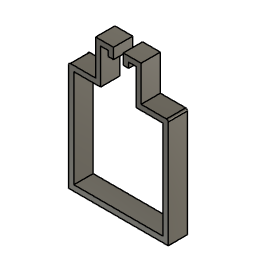
battery weight support (Autodesk Fusion 360 design; units mm, degrees)
Autodesk Fusion 360 part; units mm, degrees
sketch "Esquisse1" plane through (0, 0, 0) normal (0, 1, 0) x (1, 0, 0)
  line L0 (0, 0) -> (50, 0)
  line L1 (50, 0) -> (50, -55)
  line L2 (50, -55) -> (0, -55)
  line L3 (0, -55) -> (0, 0)
  line L4 (53, 3) -> (53, -58)
  line L5 (53, -58) -> (-3, -58)
  line L6 (-3, -58) -> (-3, 3)
  line L7 (-3, 3.2) -> (53, 3.2)
  line L8 (53, 3) -> (53, 3.2)
  line L9 (-3, 3) -> (-3, 3.2)
  line L10 (25, -55) -> (25, -58)
  line L11 (25, -58) -> (12.25, -58)
  line L12 (12.25, -58) -> (37.75, -58)
  line L13 (37.75, -58) -> (37.75, -78)
  line L14 (37.75, -78) -> (12.25, -78)
  line L15 (12.25, -78) -> (12.25, -58)
  line L16 (25, -58) -> (15, -58)
  line L17 (15, -58) -> (35, -58)
  line L18 (35, -58) -> (35, -78)
  line L19 (35, -78) -> (15, -78)
  line L20 (15, -78) -> (15, -58)
  line L21 (12.25, -58) -> (9.25, -58)
  line L22 (9.25, -58) -> (9.25, -78)
  line L23 (9.25, -78) -> (12.25, -78)
  line L24 (12.25, -78) -> (12.25, -58)
  line L25 (37.75, -58) -> (40.75, -58)
  line L26 (40.75, -58) -> (40.75, -78)
  line L27 (40.75, -78) -> (37.75, -78)
  line L28 (37.75, -78) -> (37.75, -58)
  line L29 (9.25, -78) -> (19.25, -78)
  line L30 (19.25, -78) -> (19.25, -75)
  line L31 (19.25, -75) -> (9.25, -75)
  line L32 (9.25, -75) -> (9.25, -78)
  line L33 (40.75, -78) -> (30.75, -78)
  line L34 (30.75, -78) -> (30.75, -75)
  line L35 (30.75, -75) -> (40.75, -75)
  line L36 (40.75, -75) -> (40.75, -78)
  line L37 (30.75, -75) -> (33.75, -75)
  line L38 (33.75, -75) -> (33.75, -72)
  line L39 (33.75, -72) -> (30.75, -72)
  line L40 (30.75, -72) -> (30.75, -75)
  line L41 (19.25, -75) -> (16.25, -75)
  line L42 (16.25, -75) -> (16.25, -72)
  line L43 (16.25, -72) -> (19.25, -72)
  line L44 (19.25, -72) -> (19.25, -75)
  line L45 (12.25, -58) -> (12.25, -55)
  line L46 (9.25, -58) -> (9.25, -55)
  line L47 (15, -58) -> (15, -55)
  line L48 (37.75, -58) -> (37.75, -55)
  line L49 (40.75, -58) -> (40.75, -55)
  line L50 (35, -58) -> (35, -55)
  line L51 (37.75, -78) -> (27.75, -78)
  line L52 (27.75, -78) -> (27.75, -75)
  line L53 (27.75, -75) -> (37.75, -75)
  line L54 (37.75, -75) -> (37.75, -78)
  line L55 (27.75, -75) -> (30.75, -75)
  line L56 (30.75, -75) -> (30.75, -72)
  line L57 (30.75, -72) -> (27.75, -72)
  line L58 (27.75, -72) -> (27.75, -75)
  line L59 (12.25, -78) -> (22.25, -78)
  line L60 (22.25, -78) -> (22.25, -75)
  line L61 (22.25, -75) -> (12.25, -75)
  line L62 (12.25, -75) -> (12.25, -78)
  line L63 (22.25, -75) -> (19.25, -75)
  line L64 (19.25, -75) -> (19.25, -72)
  line L65 (19.25, -72) -> (22.25, -72)
  line L66 (22.25, -72) -> (22.25, -75)
  dimension "d1" = 50
  dimension "d2" = 55
  dimension "d5" = 12.75
  dimension "d6" = 25.5
  dimension "d7" = 20
  dimension "d8" = 10
  dimension "d9" = 20
  dimension "d10" = 3
  dimension "d11" = 3
  dimension "d12" = 10
  dimension "d13" = 3
  dimension "d14" = 10
  dimension "d15" = 3
  dimension "d16" = 3
  dimension "d17" = 3
  dimension "d18" = 3
  dimension "d19" = 3
  dimension "d24" = 10
  dimension "d25" = 10
  constraint horizontal L0
  constraint vertical L1
  constraint horizontal L2
  constraint vertical L3
  constraint coincident L0.start L3.end
  constraint perpendicular L7 L8
  constraint perpendicular L7 L9
  constraint midpoint L2 L10.start
  constraint midpoint L5 L10.end
  constraint perpendicular L10 L11
  constraint horizontal L12
  constraint vertical L13
  constraint horizontal L14
  constraint vertical L15
  constraint perpendicular L10 L16
  constraint horizontal L17
  constraint vertical L18
  constraint horizontal L19
  constraint vertical L20
  constraint horizontal L21
  constraint vertical L22
  constraint horizontal L23
  constraint vertical L24
  constraint horizontal L25
  constraint vertical L26
  constraint horizontal L27
  constraint vertical L28
  constraint horizontal L29
  constraint vertical L30
  constraint horizontal L31
  constraint vertical L32
  constraint horizontal L33
  constraint vertical L34
  constraint horizontal L35
  constraint vertical L36
  constraint horizontal L37
  constraint vertical L38
  constraint horizontal L39
  constraint vertical L40
  constraint horizontal L41
  constraint vertical L42
  constraint horizontal L43
  constraint vertical L44
  constraint coincident L2 L45.end
  constraint perpendicular L2 L45
  constraint coincident L2 L46.end
  constraint perpendicular L2 L46
  constraint perpendicular L16 L47
  constraint coincident L2 L48.end
  constraint perpendicular L2 L48
  constraint perpendicular L25 L49
  constraint perpendicular L12 L50
  constraint horizontal L51
  constraint vertical L52
  constraint horizontal L53
  constraint vertical L54
  constraint horizontal L55
  constraint vertical L56
  constraint horizontal L57
  constraint vertical L58
  constraint horizontal L59
  constraint vertical L60
  constraint horizontal L61
  constraint vertical L62
  constraint horizontal L63
  constraint vertical L64
  constraint horizontal L65
  constraint vertical L66
  measures "d1" distance of L0.start L0.end
  measures "d2" distance of L0.start L2.end
  measures "d5" distance of L10.end L11.end
  measures "d6" distance of L11.end L12.end
  measures "d7" distance of L11.end L14.end
  measures "d8" distance of L10.end L16.end
  measures "d9" distance of L16.end L17.end
  measures "d10" distance of L11.end L21.end
  measures "d11" distance of L12.end L25.end
  measures "d12" distance of L22.end L29.end
  measures "d13" distance of L22.end L31.end
  measures "d14" distance of L26.end L33.end
  measures "d15" distance of L26.end L35.end
  measures "d16" distance of L34.end L37.end
  measures "d17" distance of L34.end L39.end
  measures "d18" distance of L30.end L41.end
  measures "d19" distance of L30.end L43.end
  measures "d24" distance of L13.end L51.end
  measures "d25" distance of L14.end L59.end
extrude "Extrusion1" add sketch "Esquisse1" along normal blind 10.8 contours L0 L1 L2 L3 L4 L5 L6 L7 L8 L9 L46 L49 | L2 L5 L21 L45 L46 | L2 L5 L25 L48 L49 | L2 L5 L11 L12 L45 L47 | L2 L5 L12 L48 L50 | L5 L11 L12 L15 L20 L24 L31 L61 | L5 L12 L13 L18 L28 L35 L53 | L14 L15 L20 L24 L29 L31 L59 L61 L62 | L13 L14 L18 L28 L33 L35 L51 L53 L54 | L14 L19 L20 L29 L30 L31 L41 L59 L61 | L14 L18 L19 L33 L34 L35 L37 L51 L53 | L14 L19 L30 L59 L60 L61 L63 | L44 L61 L63 L64 L65 L66 | L14 L19 L34 L51 L52 L53 L55 | L40 L53 L55 L56 L57 L58
fillet "Congé1" radius 1 2 edges at (-3, 5.4, 58) (53, 5.4, 58)
equation "d5 = ( 25.5 / 2 ) * 1 mm"
equation "d8 = ( 20 / 2 ) * 1 mm"
